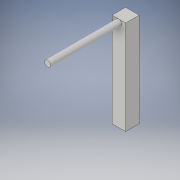
# Autodesk Inventor part: hookBoi
Saved by Autodesk Inventor 2017 (Build 210142000, 142)
## iProperties
Created: 2017-01-13
Part Number: hookBoi
Material: Generic
Document SubType Name: Modeling
Designer: kingb
Density: 1 g/cm^3
Appearance: Default
Author: kingb
Autodesk Inventor part; units mm, degrees
ref_plane "YZ Plane" through (0, 0, 0) normal (1, 0, 0) x (0, 1, 0)
ref_plane "XZ Plane" through (0, 0, 0) normal (0, 1, 0) x (-1, 0, 0)
ref_plane "XY Plane" through (0, 0, 0) normal (0, 0, 1) x (1, 0, 0)
sketch "Sketch1" plane through (0, 0, 0) normal (0, 1, 0) x (-1, 0, 0)
  line L0 (0, 0) -> (50.8, 0)
  line L1 (50.8, 0) -> (50.8, -50.8)
  line L2 (50.8, -50.8) -> (0, -50.8)
  line L3 (0, -50.8) -> (0, 0)
  dimension "d0" = 50.8
  dimension "d1" = 50.8
  constraints: 8 end point, 2 parallel, 1 horizontal, 1 perpendicular
  measures "d0" distance of L1.end L2.end
  measures "d1" distance of L0.end L1.end
extrude "Extrusion1" add sketch "Sketch1" along normal blind 352.425
sketch "Sketch2" plane through (-50.8, 0, 0) normal (0, 0, 1) x (1, 0, 0)
  line L0 (50.8, 0) -> (0, 0) projected
  line L1 (50.8, 0) -> (50.8, 352.425) projected
  line L2 (0, 352.425) -> (50.8, 352.425) projected
  line L3 (0, 0) -> (0, 352.425) projected
  line L4 (0, 352.425) -> (50.8, 352.425) construction
  circle A0 centre (25.4, 341.3125) radius 11.1125
  point P0 (25.4, 352.425)
  dimension "d6" = 11.1125
  constraints: 1 coincident, 1 midpoint, 1 vertical alignment, 2 other
  measures "d6" distance of point (25.4, 352.425) point (25.4, 341.312)
extrude "Extrusion2" add sketch "Sketch2" along normal blind 266.7 contours A0
body "Solid1"
